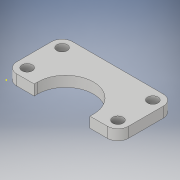
# Autodesk Inventor part: 零件2
Saved by Autodesk Inventor 2018 (Build 220112000, 112)
## iProperties
Created: 2022-10-25
Part Number: 零件2
Material: Generic
Document SubType Name: Modeling
Designer: yitxu
Density: 1 g/cm^3
Appearance: Default
Author: yitxu
Autodesk Inventor part; units mm, degrees
ref_plane "YZ Plane" through (0, 0, 0) normal (1, 0, 0) x (0, 1, 0)
ref_plane "XZ Plane" through (0, 0, 0) normal (0, 1, 0) x (-1, 0, 0)
ref_plane "XY Plane" through (0, 0, 0) normal (0, 0, 1) x (1, 0, 0)
sketch "草图1" plane through (0, 0, 0) normal (0, 1, 0) x (-1, 0, 0)
  point P0 (0, 0)
sketch "草图2" plane through (0, 0, 0) normal (0, 1, 0) x (-1, 0, 0)
  line L0 (0, 0) -> (-160, 0)
  line L1 (-160, 0) -> (-160, -80)
  line L2 (-160, -80) -> (0, -80)
  line L3 (0, -80) -> (0, 0)
  dimension "d0" = 160
  dimension "d1" = 80
  constraints: 8 end point, 2 parallel, 1 horizontal, 1 perpendicular
  measures "d0" distance of L2.end L1.end
  measures "d1" distance of L1.end L0.end
extrude "拉伸1" add sketch "草图2" along normal blind 15
fillet "圆角1" radius 15 1 edges at (160, 7.5, 0)
fillet "圆角2" radius 15 1 edges at (160, 7.5, -80)
fillet "圆角3" radius 15 1 edges at (0, 7.5, 0)
fillet "圆角4" radius 15 1 edges at (0, 7.5, -80)
sketch "草图4" plane through (0, 15, 0) normal (0, 1, 0) x (1, 0, 0)
  arc A0 (0, 15) -> (15, 0) centre (15, 15) ccw projected
  arc A1 (15, 80) -> (0, 65) centre (15, 65) ccw projected
  arc A2 (160, 65) -> (145, 80) centre (145, 65) ccw projected
  arc A3 (145, 0) -> (160, 15) centre (145, 15) ccw projected
  point P0 (0, 0)
  constraints: 4 coincident
hole "孔1" at (15, 15, -15) at (15, 15, -65) at (145, 15, -65) at (145, 15, -15) direction (0, -1, 0) diameter 15 end through all
sketch "草图5" plane through (0, 15, 0) normal (0, 1, 0) x (1, 0, 0)
  line L0 (40, 0) -> (120, 0)
  line L1 (120, 0) -> (120, 5)
  line L2 (120, 5) -> (40, 5)
  line L3 (40, 5) -> (40, 0)
  point P0 (0, 0)
  constraints: 8 end point, 3 perpendicular
extrude "拉伸2" cut sketch "草图5" against normal blind 15
sketch "草图6" plane through (0, 15, 0) normal (0, 1, 0) x (1, 0, 0)
  line L0 (120, 5) -> (40, 5) projected
  point P0 (0, 0)
  point P1 (80, 5)
  constraints: 1 midpoint
hole "孔2" at (80, 15, -5) direction (0, -1, 0) diameter 80 end through all
